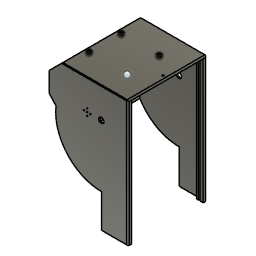
head_cover v27 (Autodesk Fusion 360 design; units mm, degrees)
Autodesk Fusion 360 part; units mm, degrees
note: some values were not read from the file. Set by a fixed rule: which sketch regions a step uses.
sketch "Sketch1" plane through (0, 0, 0) normal (0, 1, 0) x (1, 0, 0)
  line L0 (20, -60) -> (120, -60)
  line L1 (120, -60) -> (120, 0)
  line L2 (0, -10) -> (0, -40)
  line L3 (10.4331, 1.3041) -> (10.5405, 1.3176)
  line L4 (80, 80) -> (80, 132)
  line L5 (80, 132) -> (120, 132)
  line L6 (120, 132) -> (120, 0)
  line L7 (0, -40) -> (20, -60)
  line L8 (0, -10) -> (10.4331, 1.3041)
  arc A0 (80, 80) -> (10.5405, 1.3176) centre (80, 10) ccw
  dimension "d2" = 60
  dimension "d3" = 132
  dimension "d6" = 15.3829
  dimension "d7" = 30
  dimension "d8" = 28.2843
  dimension "d9" = 100
  dimension "d10" = 40
  dimension "d48" = 70
  constraint horizontal L0
  constraint vertical L1
  constraint vertical L2
  constraint vertical L4
  constraint horizontal L5
  constraint vertical L6
  measures "d2" distance of L0.end L1.end
  measures "d3" distance of L1.end L5.end
  measures "d6" distance of L2.start L3.start
  measures "d7" distance of L2.end L2.start
  measures "d8" distance of L2.end L0.start
  measures "d9" distance of L0.end L0.start
  measures "d10" distance of L4.end L5.end
  measures "d48" radius of A0
extrude "Extrude1" add sketch "Sketch1" along normal blind 120.4
sketch "Sketch3" plane through (120, 0, 0) normal (1, 0, 0) x (0, 1, 0)
  line L0 (0, 60) -> (0, -132)
  line L1 (0, -132) -> (120.4, -132)
  line L2 (120.4, -132) -> (120.4, 60)
  line L3 (120.4, 60) -> (0, 60)
  line L4 (2.1, 57.9) -> (118.3, 57.9)
  line L5 (118.3, 57.9) -> (118.3, -56)
  line L6 (2.1, -56) -> (2.1, 57.9)
  line L7 (2.1, -56) -> (2.1, -132)
  line L8 (118.3, -132) -> (118.3, -56)
  dimension "d14" = 2.1
  dimension "d15" = 2.1
  dimension "d16" = 2.1
  dimension "d19" = 2.1
  dimension "d20" = 2.1
  constraint horizontal L4
  constraint vertical L5
  constraint vertical L6
  constraint coincident L1 L7.end
  constraint perpendicular L1 L7
  constraint coincident L1 L8.start
  measures "d14" distance of L3 L4
  measures "d15" distance of L0 L6
  measures "d16" distance of L2 L5
  measures "d19" distance of L0 L7
  measures "d20" distance of L2 L8
extrude "Extrude2" cut sketch "Sketch3" against normal blind 100 contours L1 L4 L5 L6 L7 L8
sketch "Sketch5" plane through (0, 0, 57.9) normal (0, 0, -1) x (1, 0, 0)
  line L0 (120, -118.3) -> (120, -2.1)
  line L1 (20, -2.1) -> (20, -118.3)
  line L2 (20, -118.3) -> (120, -118.3)
  line L3 (120, -118.3) -> (112.8, -118.3)
  line L4 (112.8, -118.3) -> (112.8, -2.1)
  line L5 (112.8, -2.1) -> (120, -2.1)
  line L6 (120, -2.1) -> (120, -118.3)
  line L7 (120, -2.1) -> (20, -2.1)
  dimension "d24" = 7.2
  constraint horizontal L3
  constraint vertical L4
  constraint horizontal L5
  constraint vertical L6
  constraint coincident L0.start L2.end
  measures "d24" distance of L4.end L0.end
extrude "Extrude3" cut sketch "Sketch5" against normal blind 2.5 contours L0 L2 L3 L4 L5 L6 L7
sketch "Sketch7" plane through (0, 2.1, 0) normal (0, 1, 0) x (-1, 0, 0)
  line L0 (-80, -132) -> (-80, -80)
  line L1 (-20, -46.0555) -> (-20, 57.9)
  line L2 (-20, 57.9) -> (-112.8, 57.9)
  line L3 (-112.8, 57.9) -> (-112.8, 60)
  line L4 (-112.8, 60) -> (-120, 60)
  line L5 (-120, 60) -> (-120, -132)
  line L6 (-120, -132) -> (-80, -132)
  line L7 (-112, 57.9) -> (-120, 57.9)
  line L8 (-120, 57.9) -> (-120, -132)
  line L9 (-120, -132) -> (-112, -132)
  line L10 (-112, -132) -> (-112, 57.9)
  arc A0 (-80, -80) -> (-20, -46.0555) centre (-80, -10) ccw
  dimension "d27" = 8
  constraint horizontal L7
  constraint vertical L8
  constraint horizontal L9
  constraint vertical L10
  constraint coincident L5.end L6.start
  constraint coincident L2 L7.start
  measures "d27" distance of L5.end L9.end
extrude "Extrude4" add sketch "Sketch7" along normal blind 3.6 contours L2 L5 L6 L7 L8 L9 L10
sketch "Sketch8" plane through (0, 0, 57.9) normal (0, 0, 1) x (-1, 0, 0)
  line L0 (-112.8, -5.7) -> (-112.8, -2.1)
  line L1 (-112.8, -2.1) -> (-120, -2.1)
  line L2 (-120, -2.1) -> (-120, -5.7)
  line L3 (-120, -5.7) -> (-112.8, -5.7)
  line L4 (-112.8, -2.1) -> (-115.3, -2.1)
  line L5 (-115.3, -2.1) -> (-115.3, -5.7)
  line L6 (-115.3, -5.7) -> (-112.8, -5.7)
  line L7 (-112.8, -5.7) -> (-112.8, -2.1)
  dimension "d30" = 2.5
  constraint horizontal L4
  constraint vertical L5
  constraint horizontal L6
  constraint vertical L7
  constraint coincident L3 L5.end
  constraint coincident L0.end L1.start
  measures "d30" distance of L5.end L0.start
extrude "Extrude5" cut sketch "Sketch8" against normal blind 190 contours L0 L1 L3 L4 L5 L6 L7
sketch "Sketch9" plane through (0, 118.3, 0) normal (0, -1, 0) x (1, 0, 0)
  line L0 (80, -80) -> (80, -132)
  line L1 (80, -132) -> (120, -132)
  line L2 (120, -132) -> (120, 60)
  line L3 (120, 60) -> (112.8, 60)
  line L4 (112.8, 60) -> (112.8, 57.9)
  line L5 (112.8, 57.9) -> (20, 57.9)
  line L6 (20, 57.9) -> (20, -46.0555)
  line L7 (112, 57.9) -> (120, 57.9)
  line L8 (120, 57.9) -> (120, -132)
  line L9 (120, -132) -> (112, -132)
  line L10 (112, -132) -> (112, 57.9)
  arc A0 (20, -46.0555) -> (80, -80) centre (80, -10) ccw
  dimension "d33" = 8
  constraint horizontal L7
  constraint vertical L8
  constraint horizontal L9
  constraint vertical L10
  constraint coincident L1.end L2.start
  constraint coincident L5 L7.start
  measures "d33" distance of L1.end L9.end
extrude "Extrude6" add sketch "Sketch9" along normal blind 3.6 contours L1 L2 L5 L7 L8 L9 L10
sketch "Sketch10" plane through (0, 0, 57.9) normal (0, 0, 1) x (-1, 0, 0)
  line L0 (-112.8, -118.3) -> (-112.8, -114.7)
  line L1 (-112.8, -114.7) -> (-120, -114.7)
  line L2 (-120, -114.7) -> (-120, -118.3)
  line L3 (-120, -118.3) -> (-112.8, -118.3)
  line L4 (-112.8, -118.3) -> (-115.3, -118.3)
  line L5 (-115.3, -118.3) -> (-115.3, -114.7)
  line L6 (-115.3, -114.7) -> (-112.8, -114.7)
  line L7 (-112.8, -114.7) -> (-112.8, -118.3)
  dimension "d36" = 2.5
  constraint horizontal L4
  constraint vertical L5
  constraint horizontal L6
  constraint vertical L7
  constraint coincident L1 L5.end
  constraint coincident L0.start L3.end
  measures "d36" distance of L0.start L4.end
extrude "Extrude7" cut sketch "Sketch10" against normal blind 190 contours L0 L1 L3 L4 L5 L6 L7
chamfer "Chamfer1" distance 1 angle 45 4 edges at (100, 0, -132) (100, 120.4, -132) (70, 0, 60) (70, 120.4, 60)
sketch "Sketch15" plane through (112.8, 0, 0) normal (1, 0, 0) x (0, 1, 0)
  line L0 (118.3, 60) -> (2.1, 60)
  line L1 (2.1, 60) -> (2.1, -132)
  line L2 (5.7, -132) -> (5.7, 57.9)
  line L3 (5.7, 57.9) -> (114.7, 57.9)
  line L4 (114.7, 57.9) -> (114.7, -132)
  line L5 (118.3, -132) -> (118.3, 60)
  line L6 (2.1, 60) -> (118.3, 60)
  line L7 (118.3, 60) -> (118.3, 57.9)
  line L8 (118.3, 57.9) -> (2.1, 57.9)
  line L9 (2.1, 57.9) -> (2.1, 60)
  line L10 (2.1, -132) -> (5.7, -132)
  line L11 (114.7, -132) -> (118.3, -132)
  constraint horizontal L6
  constraint vertical L7
  constraint horizontal L8
  constraint vertical L9
  constraint coincident L5 L7.end
  constraint coincident L0.end L1.start
extrude "Extrude11" add sketch "Sketch15" along normal blind 7.2 contours L0 L1 L3 L5 L6 L7 L8 L9
sketch "Sketch16" plane through (0, 2.1, 0) normal (0, 1, 0) x (-1, 0, 0)
  line L0 (-112, 57.9) -> (-112, -132)
  line L1 (-112, -132) -> (-80, -132)
  line L2 (-80, -132) -> (-80, -80)
  arc A0 (-80, -80) -> (-20, -46.0555) centre (-80, -10) ccw
  line L3 (-20, -46.0555) -> (-20, 57.9)
  line L4 (-20, 57.9) -> (-112, 57.9)
  line L5 (-112, 57.9) -> (-110, 57.9)
  line L6 (-110, 57.9) -> (-110, -132)
  line L7 (-110, -132) -> (-112, -132)
  line L8 (-112, -132) -> (-112, 57.9)
  dimension "d54" = 2
  constraint horizontal L5
  constraint vertical L6
  constraint horizontal L7
  constraint vertical L8
  constraint coincident L1 L6.end
  constraint coincident L0.start L4.end
  measures "d54" distance of L6 L8
extrude "Extrude12" add sketch "Sketch16" along normal blind 3.6 contours L0 L1 L4 L5 L6 L7 L8
sketch "Sketch17" plane through (0, 118.3, 0) normal (0, -1, 0) x (1, 0, 0)
  line L0 (112, -132) -> (112, 57.9)
  line L1 (112, 57.9) -> (20, 57.9)
  line L2 (20, 57.9) -> (20, -46.0555)
  arc A0 (20, -46.0555) -> (80, -80) centre (80, -10) ccw
  line L3 (80, -80) -> (80, -132)
  line L4 (80, -132) -> (112, -132)
  line L5 (112, 57.9) -> (110, 57.9)
  line L6 (110, 57.9) -> (110, -132)
  line L7 (110, -132) -> (112, -132)
  line L8 (112, -132) -> (112, 57.9)
  dimension "d57" = 2
  constraint horizontal L5
  constraint vertical L6
  constraint horizontal L7
  constraint vertical L8
  constraint coincident L4 L6.end
  constraint coincident L0.end L1.start
  measures "d57" distance of L6 L8
extrude "Extrude13" add sketch "Sketch17" along normal blind 3.6 contours L0 L1 L4 L5 L6 L7 L8
sketch "Sketch18" plane through (0, 0, 57.9) normal (0, 0, -1) x (1, 0, 0)
  line L0 (110, -118.3) -> (110, -114.7)
  line L1 (110, -114.7) -> (112.8, -114.7)
  line L2 (112.8, -114.7) -> (112.8, -118.3)
  line L3 (112.8, -118.3) -> (115.3, -118.3)
  line L4 (115.3, -118.3) -> (115.3, -114.7)
  line L5 (115.3, -114.7) -> (120, -114.7)
  line L6 (120, -114.7) -> (120, -5.7)
  line L7 (120, -5.7) -> (115.3, -5.7)
  line L8 (115.3, -5.7) -> (115.3, -2.1)
  line L9 (115.3, -2.1) -> (112.8, -2.1)
  line L10 (112.8, -2.1) -> (112.8, -5.7)
  line L11 (112.8, -5.7) -> (110, -5.7)
  line L12 (110, -5.7) -> (110, -2.1)
  line L13 (110, -2.1) -> (20, -2.1)
  line L14 (20, -2.1) -> (20, -118.3)
  line L15 (20, -118.3) -> (110, -118.3)
  circle A0 centre (25, -84.8) radius 2.5
  circle A1 centre (25, -35.8) radius 2.5
  circle A2 centre (83, -35.8) radius 2.5
  circle A3 centre (83, -84.8) radius 2.5
  circle A4 centre (83, -35.8) radius 1.375
  circle A5 centre (25, -35.8) radius 1.375
  circle A6 centre (83, -84.8) radius 1.375
  circle A7 centre (25, -84.8) radius 1.375
  dimension "d60" = 5
  dimension "d61" = 5
  dimension "d62" = 49
  dimension "d63" = 49
  dimension "d64" = 58
  dimension "d65" = 33.5
  dimension "d66" = 33.5
  dimension "d67" = 5
  dimension "d68" = 5
  dimension "d71" = 2.75
  dimension "d72" = 2.75
  dimension "d73" = 2.75
  dimension "d74" = 2.75
  dimension "d77" = 5
  dimension "d78" = 58
  dimension "d79" = 5
  constraint concentric A2 A4
  constraint concentric A1 A5
  constraint concentric A3 A6
  constraint concentric A0 A7
  measures "d60" diameter of A0
  measures "d61" diameter of A1
  measures "d62" distance of A0.centre A1.centre
  measures "d63" distance of A2.centre A3.centre
  measures "d64" horizontal distance of A0.centre A3.centre
  measures "d65" distance of L15 A3.centre
  measures "d66" distance of L15 A0.centre
  measures "d67" diameter of A3
  measures "d68" diameter of A2
  measures "d71" diameter of A5
  measures "d72" diameter of A4
  measures "d73" diameter of A6
  measures "d74" diameter of A7
  measures "d77" distance of L14 A1.centre
  measures "d78" distance of A1.centre A2.centre
  measures "d79" distance of L14 A0.centre
extrude "Extrude15" add sketch "Sketch18" along normal blind 5 contours A0 | A1 | A2 | A3
chamfer "Chamfer2" distance 2 angle 45 3 edges at (120, 60.2, 60) (120, 0, -36) (120, 120.4, -36)
sketch "Sketch19" plane through (0, 120.4, 0) normal (0, 1, 0) x (-1, 0, 0)
  line L0 (-118, 59) -> (-118, -131)
  line L1 (-118, -131) -> (-80, -131)
  line L2 (-80, -131) -> (-80, -80)
  arc A0 (-80, -80) -> (-10.5405, -1.3176) centre (-80, -10) ccw
  line L3 (-10.5405, -1.3176) -> (-10.4331, -1.3041)
  line L4 (-10.4331, -1.3041) -> (0, 10)
  line L5 (0, 10) -> (0, 40)
  line L6 (0, 40) -> (-19, 59)
  line L7 (-19, 59) -> (-118, 59)
  circle A1 centre (-50, 14) radius 1
  circle A2 centre (-50, 19) radius 1
  circle A3 centre (-45, 14) radius 1
  circle A4 centre (-55, 14) radius 1
  circle A5 centre (-50, 9) radius 1
  line L8 (-110, 57.9) -> (-110, -132)
  dimension "d81" = 2
  dimension "d82" = 2
  dimension "d83" = 2
  dimension "d84" = 2
  dimension "d85" = 2
  dimension "d86" = 5
  dimension "d87" = 5
  dimension "d88" = 5
  dimension "d89" = 5
  dimension "d90" = 60
  dimension "d93" = 45
  measures "d81" diameter of A1
  measures "d82" diameter of A2
  measures "d83" diameter of A3
  measures "d84" diameter of A4
  measures "d85" diameter of A5
  measures "d86" distance of A1.centre A4.centre
  measures "d87" distance of A1.centre A3.centre
  measures "d88" distance of A1.centre A2.centre
  measures "d89" distance of A1.centre A5.centre
  measures "d90" distance of A1.centre L8
  measures "d93" distance of L7 A1.centre
extrude "Extrude16" cut sketch "Sketch19" against normal blind 5 contours A1 | A2 | A3 | A4 | A5
sketch "Sketch20" plane through (0, 0, 0) normal (0, -1, 0) x (1, 0, 0)
  line L0 (118, -131) -> (118, 59)
  line L1 (118, 59) -> (19, 59)
  line L2 (19, 59) -> (0, 40)
  line L3 (0, 40) -> (0, 10)
  line L4 (0, 10) -> (10.4331, -1.3041)
  line L5 (10.4331, -1.3041) -> (10.5405, -1.3176)
  arc A0 (10.5405, -1.3176) -> (80, -80) centre (80, -10) ccw
  line L6 (80, -80) -> (80, -131)
  line L7 (80, -131) -> (118, -131)
  circle A1 centre (58, 14) radius 1
  circle A2 centre (58, 19) radius 1
  circle A3 centre (63, 14) radius 1
  circle A4 centre (53, 14) radius 1
  circle A5 centre (58, 9) radius 1
  dimension "d94" = 2
  dimension "d95" = 2
  dimension "d96" = 2
  dimension "d97" = 2
  dimension "d98" = 2
  dimension "d99" = 5
  dimension "d100" = 5
  dimension "d101" = 5
  dimension "d102" = 5
  dimension "d103" = 60
  dimension "d104" = 45
  measures "d94" diameter of A1
  measures "d95" diameter of A2
  measures "d96" diameter of A3
  measures "d97" diameter of A4
  measures "d98" diameter of A5
  measures "d99" distance of A1.centre A5.centre
  measures "d100" distance of A1.centre A3.centre
  measures "d101" distance of A1.centre A4.centre
  measures "d102" distance of A1.centre A2.centre
  measures "d103" distance of L0 A1.centre
  measures "d104" distance of L1 A1.centre
extrude "Extrude17" cut sketch "Sketch20" against normal blind 5 contours A1 | A2 | A3 | A4 | A5
sketch "Sketch21" plane through (0, 0, 0) normal (0, -1, 0) x (1, 0, 0)
  circle A0 centre (58, 9) radius 1
  circle A1 centre (63, 14) radius 1
  circle A2 centre (53, 14) radius 1
  circle A3 centre (58, 19) radius 1
  circle A4 centre (58, 14) radius 1
  line L0 (118, -131) -> (118, 59)
  line L1 (118, 59) -> (19, 59)
  line L2 (19, 59) -> (0, 40)
  line L3 (0, 40) -> (0, 10)
  line L4 (0, 10) -> (10.4331, -1.3041)
  line L5 (10.4331, -1.3041) -> (10.5405, -1.3176)
  arc A5 (10.5405, -1.3176) -> (80, -80) centre (80, -10) ccw
  line L6 (80, -80) -> (80, -131)
  line L7 (80, -131) -> (118, -131)
  circle A6 centre (79.5207, 14) radius 4.025
  dimension "d107" = 8.05
  measures "d107" diameter of A6
extrude "Extrude18" cut sketch "Sketch21" against normal blind 170 contours A6
sketch "Sketch22" plane through (0, 0, 60) normal (0, 0, 1) x (-1, 0, 0)
  line L0 (-118, -1) -> (-118, -119.4)
  line L1 (-118, -119.4) -> (-20, -119.4)
  line L2 (-20, -119.4) -> (-20, -1)
  line L3 (-20, -1) -> (-118, -1)
  circle A0 centre (-113.6, -60.2) radius 1.375
  dimension "d110" = 4.4
  dimension "d111" = 2.75
  dimension "d112" = 59.2
  measures "d110" distance of L0 A0.centre
  measures "d111" diameter of A0
  measures "d112" distance of L3 A0.centre
extrude "Extrude19" cut sketch "Sketch22" against normal blind 3 contours A0
